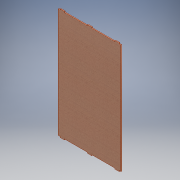
# Autodesk Inventor part: Superior_top
Saved by Autodesk Inventor 2017 (Build 210142000, 142)
## iProperties
Created: 2017-10-02
Part Number: Superior_top
Material: Wood (Oak)
Document SubType Name: Modeling
Designer: Felipe
Density: 0.76 g/cm^3
Appearance: White Oak - Natural Medium Gloss
Author: Felipe
Autodesk Inventor part; units mm, degrees
ref_plane "YZ Plane" through (0, 0, 0) normal (1, 0, 0) x (0, 1, 0)
ref_plane "XZ Plane" through (0, 0, 0) normal (0, 1, 0) x (-1, 0, 0)
ref_plane "XY Plane" through (0, 0, 0) normal (0, 0, 1) x (1, 0, 0)
sketch "Sketch1" plane through (0, 0, 0) normal (0, 1, 0) x (-1, 0, 0)
  line L0 (0, 0) -> (515, 0) construction
  line L1 (515, 0) -> (515, -900)
  line L2 (515, -900) -> (0, -900) construction
  line L3 (0, -900) -> (0, 0)
  line L4 (500, 0) -> (465, 0) construction
  line L5 (465, 0) -> (465, 7.3489)
  line L6 (465, 7.3489) -> (500, 7.3489)
  line L7 (500, 7.3489) -> (500, 0)
  line L8 (275, 0) -> (240, 0) construction
  line L9 (240, 0) -> (240, 7.3489)
  line L10 (240, 7.3489) -> (275, 7.3489)
  line L11 (275, 7.3489) -> (275, 0)
  line L12 (515, 0) -> (500, 0)
  line L13 (0, 0) -> (240, 0) construction
  line L14 (465, 0) -> (275, 0)
  line L15 (0, -450) -> (515, -450) construction
  line L16 (465, -900) -> (465, -907.3489)
  line L17 (465, -907.3489) -> (500, -907.3489)
  line L18 (500, -907.3489) -> (500, -900)
  line L19 (240, -900) -> (240, -907.3489)
  line L20 (240, -907.3489) -> (275, -907.3489)
  line L21 (275, -907.3489) -> (275, -900)
  line L22 (0, -900) -> (240, -900) construction
  line L23 (275, -900) -> (465, -900)
  line L24 (500, -900) -> (515, -900)
  line L25 (50, 0) -> (15, 0) construction
  line L26 (15, 0) -> (15, 7.3489)
  line L27 (15, 7.3489) -> (50, 7.3489)
  line L28 (50, 7.3489) -> (50, 0)
  line L29 (240, 0) -> (50, 0)
  line L30 (15, 0) -> (0, 0)
  line L31 (50, -900) -> (15, -900) construction
  line L32 (15, -900) -> (15, -907.3489)
  line L33 (15, -907.3489) -> (50, -907.3489)
  line L34 (50, -907.3489) -> (50, -900)
  line L35 (240, -900) -> (50, -900)
  line L36 (15, -900) -> (0, -900)
  dimension "d0" = 900
  dimension "d1" = 515
  dimension "d4" = 35
  dimension "d5" = 35
  dimension "d6" = 190
  dimension "d7" = 15
  dimension "d8" = 240
  dimension "d9" = 190
  constraints: 74 end point, 12 symmetric about line, 8 collinear, 8 parallel, 6 perpendicular, 5 point on line, 4 horizontal, 2 equal length, 2 midpoint
  measures "d0" distance of L0.end L1.end
  measures "d1" distance of L0.start L0.end
  measures "d4" distance of L5.end L6.end
  measures "d5" distance of L9.end L10.end
  measures "d6" distance between parallel lines of L5 L11
  measures "d7" distance between parallel lines of L1 L7
  measures "d8" distance between parallel lines of L3 L9
  measures "d9" distance between parallel lines of L28 L9
extrude "Extrusion1" add sketch "Sketch1" along normal blind 6
body "Solid1"
